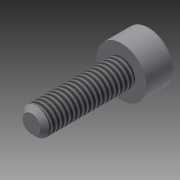
# Autodesk Inventor part: M3x10SHCS
Saved by Autodesk Inventor 2016 (Build 200138000, 138)
## iProperties
Category: Hardware
Created: 2013-12-15
Part Number: M3x10SHCS
Material: Generic
Document SubType Name: Modeling
Designer: Jack
Density: 1 g/cm^3
Appearance: Default
Vendor: McMaster Carr
Stock Number: CB3-10
Mass: 0.130088 g
Surface Area: 2.07835 cm^2
Volume: 0.130088 cm^3
Author: Jack
Title: SHCS 3x10
Autodesk Inventor part; units mm, degrees
ref_plane "YZ Plane" through (0, 0, 0) normal (1, 0, 0) x (0, 1, 0)
ref_plane "XZ Plane" through (0, 0, 0) normal (0, 1, 0) x (-1, 0, 0)
ref_plane "XY Plane" through (0, 0, 0) normal (0, 0, 1) x (1, 0, 0)
sketch "Sketch1" plane through (0, 0, 0) normal (0, 1, 0) x (-1, 0, 0)
  circle A0 centre (0, 0) radius 1.5
  dimension "d0" = 3
  constraints: 1 centre point, 1 coincident
  measures "d0" diameter of A0
extrude "Extrusion1" add sketch "Sketch1" along normal blind 10
sketch "Sketch2" plane through (0, 10, 0) normal (0, 1, 0) x (1, 0, 0)
  circle A0 centre (0, 0) radius 1.5 projected
  circle A1 centre (0, 0) radius 2.75
  dimension "d3" = 5.5
  constraints: 1 centre point, 1 coincident
  measures "d3" diameter of A1
extrude "Extrusion2" add sketch "Sketch2" along normal blind 3 contours A0 | A1
sketch "Sketch3" plane through (0, 13, 0) normal (0, 1, 0) x (1, 0, 0)
  circle A0 centre (0, 0) radius 2.75 projected
  line L0 (0, 1.4434) -> (1.25, 0.7217)
  line L1 (1.25, 0.7217) -> (1.25, -0.7217)
  line L2 (1.25, -0.7217) -> (0, -1.4434)
  line L3 (0, -1.4434) -> (-1.25, -0.7217)
  line L4 (-1.25, -0.7217) -> (-1.25, 0.7217)
  line L5 (-1.25, 0.7217) -> (0, 1.4434)
  dimension "d6" = 2.5
  constraints: 12 end point, 1 coincident, 1 vertical, 13 other
  measures "d6" distance between parallel lines of L1 L4
extrude "Extrusion3" cut sketch "Sketch3" against normal blind 2 contours L0 L1 L2 L3 L4 L5
thread "Thread1" size "M3x0.5" class "6g" standard "ANSI Metric M Profile" full length
chamfer "Chamfer1" distance 0.5 angle 45 1 edges at (1.5, 0, 0)
body "Solid1"
